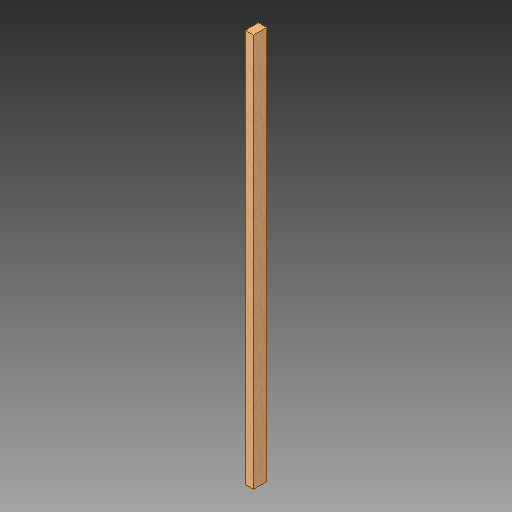
# Autodesk Inventor part: feet
Saved by Autodesk Inventor 2019 (Build 230136000, 136)
## iProperties
Created: 2019-05-05
Part Number: feet
Material: Madeira
Document SubType Name: Modeling
Designer: Daniel Regner
Density: 0.570257 g/cm^3
Appearance: Pinho amarelo - Sólido natural sem brilho
lenght: 25,000 mm
widht: 40,000 mm
Author: Daniel Regner
Autodesk Inventor part; units mm, degrees
ref_plane "YZ Plane" through (0, 0, 0) normal (1, 0, 0) x (0, 1, 0)
ref_plane "XZ Plane" through (0, 0, 0) normal (0, 1, 0) x (-1, 0, 0)
ref_plane "XY Plane" through (0, 0, 0) normal (0, 0, 1) x (1, 0, 0)
sketch "Esboço1" plane through (0, 0, 0) normal (0, 1, 0) x (-1, 0, 0)
  line L0 (-12.5, 20) -> (12.5, 20)
  line L1 (12.5, 20) -> (12.5, -20)
  line L2 (12.5, -20) -> (-12.5, -20)
  line L3 (-12.5, -20) -> (-12.5, 20)
  line L4 (-12.5, 20) -> (12.5, -20) construction
  line L5 (12.5, 20) -> (-12.5, -20) construction
  point P0 (0, 0)
  dimension "lenght" = 25
  dimension "widht" = 40
  constraints: 12 end point, 2 midpoint, 2 parallel, 1 horizontal, 1 perpendicular
  measures "lenght" distance of L1.end L2.end
  measures "widht" distance of L0.end L1.end
extrude "Extrusão1" add sketch "Esboço1" along normal mid plane 1200
equation "\"lenght\" = RIP_L"
equation "\"widht\" = RIP_H"
equation "\"d2\" = HEIGHT"
equation "\"HEIGHT\" = 1200"
equation "\"RIP_H\" = 40"
equation "\"RIP_L\" = 25"
